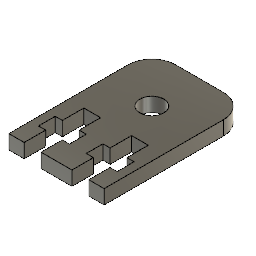
stand_R v3 (Autodesk Fusion 360 design; units mm, degrees)
Autodesk Fusion 360 part; units mm, degrees
note: some values were not read from the file. Set by a fixed rule: which sketch regions a step uses.
sketch "Sketch1" plane through (0, 0, 0) normal (0, 0, 1) x (1, 0, 0)
  line L0 (0, 0) -> (40, 0)
  line L1 (40, 0) -> (40, 60)
  line L2 (40, 60) -> (0, 60)
  line L3 (0, 60) -> (0, 0)
  line L4 (20, 60) -> (20, 27.089)
  circle A0 centre (20, 40) radius 5
  line L5 (6.5, 0) -> (13.5, 0)
  line L6 (13.5, 0) -> (13.5, 25)
  line L7 (13.5, 25) -> (6.5, 25)
  line L8 (6.5, 25) -> (6.5, 0)
  line L9 (26.5, 0) -> (33.5, 0)
  line L10 (33.5, 0) -> (33.5, 25)
  line L11 (33.5, 25) -> (26.5, 25)
  line L12 (26.5, 25) -> (26.5, 0)
  line L13 (10, 25) -> (30, 25)
  line L14 (20, 25) -> (20, 0)
  line L15 (0, 16) -> (40, 16)
  line L16 (3.5, 16) -> (16.5, 16)
  line L17 (16.5, 16) -> (16.5, 9)
  line L18 (16.5, 9) -> (3.5, 9)
  line L19 (3.5, 9) -> (3.5, 16)
  line L20 (3.5, 12.5) -> (6.5, 12.5)
  line L21 (10, 9) -> (10, 0)
  line L22 (23.5, 16) -> (23.5, 9)
  line L23 (23.5, 9) -> (36.5, 9)
  line L24 (36.5, 9) -> (36.5, 16)
  dimension "d1" = 40
  dimension "d2" = 60
  dimension "d3" = 10
  dimension "d4" = 40
  dimension "d5" = 7
  dimension "d6" = 7
  dimension "d7" = 25
  dimension "d8" = 25
  dimension "d9" = 20
  dimension "d10" = 90
  dimension "d11" = 90
  dimension "d12" = 13
  dimension "d13" = 90
  dimension "d14" = 7
  constraint horizontal L0
  constraint vertical L1
  constraint horizontal L2
  constraint vertical L3
  constraint coincident L0.start L3.end
  constraint midpoint L2 L4.start
  constraint perpendicular L2 L4
  constraint coincident L4 A0.centre
  constraint horizontal L5
  constraint vertical L6
  constraint horizontal L7
  constraint vertical L8
  constraint coincident L0 L5.start
  constraint horizontal L9
  constraint vertical L10
  constraint horizontal L11
  constraint vertical L12
  constraint coincident L0 L9.start
  constraint midpoint L7 L13.start
  constraint midpoint L11 L13.end
  constraint midpoint L13 L14.start
  constraint midpoint L0 L14.end
  constraint coincident L3 L15.start
  constraint coincident L1 L15.end
  constraint perpendicular L1 L15
  constraint horizontal L16
  constraint vertical L17
  constraint horizontal L18
  constraint vertical L19
  constraint coincident L15 L16.start
  constraint midpoint L19 L20.start
  constraint midpoint L8 L20.end
  constraint midpoint L18 L21.start
  constraint midpoint L5 L21.end
  constraint symmetric L14 L16.start L24.end
  constraint symmetric L14 L16.end L22.start
  constraint symmetric L14 L17.end L22.end
  constraint symmetric L14 L18.end L23.end
  measures "d1" distance of L0.start L0.end
  measures "d2" distance of L0.end L1.end
  measures "d3" diameter of A0
  measures "d4" distance of L0 A0.centre
  measures "d5" distance of L6.end L7.end
  measures "d6" distance of L10.end L11.end
  measures "d7" distance of L5.start L7.end
  measures "d8" distance of L9.end L10.end
  measures "d9" distance of L13.start L13.end
  measures "d10" angle of L0 L14
  measures "d11" angle of L8 L20
  measures "d12" distance of L17.end L18.end
  measures "d13" angle of L18 L21 L9.start
  measures "d14" distance of L16.end L17.end
extrude "Extrude1" add sketch "Sketch1" along normal blind 6 contours L0 L3 L8 L15 L18 L19 | L1 L2 L3 L7 L8 L10 L11 L13 L15 L16 | L0 L6 L14 L15 L17 L18 | L0 L12 L14 L15 L22 L23 | L6 L13 L14 L15 L16 | L12 L13 L14 L15 | L0 L1 L10 L15 L23 L24
fillet "Fillet1" radius 10 1 edges at (0, 60, 3)
fillet "Fillet2" radius 10 1 edges at (40, 60, 3)
